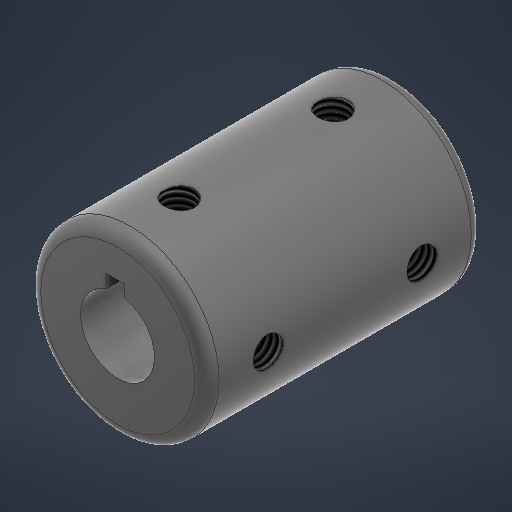
# Autodesk Inventor part: Accouplement12-12
Saved by Autodesk Inventor 2026.2 (Build 302298010, 298A)
## iProperties
Created: 2026-04-18
Part Number: Accouplement12-12
Material: Générique
Document SubType Name: Modeling
Designer: romai
Density: 1 g/cm^3
Appearance: Par défaut
Author: romai
Autodesk Inventor part; units mm, degrees
note: some values were not read from the file. Chosen so that the rebuilt part matches the saved one: direction of "Perçage1".
sketch "Esquisse1" plane through (0, 0, 0) normal (0, 0, 1) x (1, 0, 0)
  circle A0 centre (0, 0) radius 6
  circle A1 centre (0, 0) radius 14.5
  line L0 (-1.8, 7.8788) -> (1.1996, 7.8788)
  line L1 (1.1996, 7.8788) -> (1.1996, 6)
  line L2 (1.1996, 6) -> (0, 6)
  line L3 (-1.8, 5.9539) -> (-1.8, 7.8788)
  line L4 (0, 5.8848) -> (1.1996, 6) construction
  line L5 (1.1996, 7.8788) -> (0, 5.8848) construction
  line L6 (-1.8, 5.9539) -> (-1.8, 5.7236)
  line L7 (1.1996, 6) -> (1.1996, 5.8788)
  dimension "d0" = 12
  dimension "d1" = 29
  dimension "d2" = 3
  dimension "d3" = 2
  dimension "d4" = 0
  constraints: 16 end point, 3 parallel, 3 point on circle, 2 centre point, 2 coincident, 1 horizontal, 1 perpendicular, 1 tangent, 1 vertical
  measures "d0" diameter of A0
  measures "d1" diameter of A1
  measures "d2" distance of L1.end L3.start
  measures "d3" distance of L7.end L0.end
  measures "d4" horizontal distance of L4.start L2.end
extrude "Extrusion1" add sketch "Esquisse1" against normal blind 45
fillet "Congé1" radius 2 2 edges at (-14.5, 0, 0) (-14.5, 0, -45)
ref_plane "Plan de construction1" through (14.5, 0, 0) normal (1, 0, 0) x (0, 0, -1)
sketch "Esquisse2" plane through (14.5, 0, 0) normal (1, 0, 0) x (0, 0, -1)
  point P0 (0, 0)
  point P1 (10, -0.1022)
  dimension "d15" = 10
  measures "d15" horizontal distance of point (0, 0) point (10, -0.102)
hole "Perçage1" at (14.5, -0.1022, -10) direction (-1, 0, 0) diameter 4.917 end up to surface thread size "M6x1" class "6H" standard "ISO Metric profile"
ref_plane "Plan de construction2" through (0, 14.5, 0) normal (0, -1, 0) x (1, 0, 0)
sketch "Esquisse3" plane through (0, 14.5, 0) normal (0, -1, 0) x (1, 0, 0)
  point P0 (0, 0)
  point P1 (0.0163, -10)
  dimension "d23" = 10
  measures "d23" distance of point (0, 0) point (0.016, -10)
hole "Perçage2" at (0.0163, 14.5, -10) direction (0, -1, 0) diameter 4.917 end up to surface thread size "M6x1" class "6H" standard "ISO Metric profile"
ref_plane "Plan de construction3" through (0, 0, -22.5) normal (0, 0, 1) x (1, 0, 0)
mirror "Mise en miroir1" about plane through (0, 0, -22.5) normal (0, 0, 1) of "Perçage2", "Perçage1"
